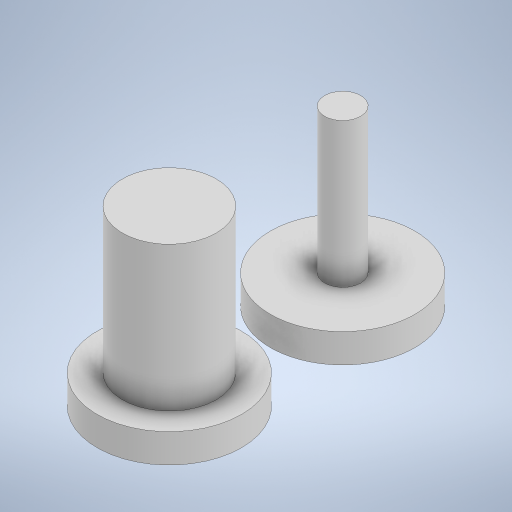
# Autodesk Inventor part: V3_O1
Saved by Autodesk Inventor 2023.1 (Build 271208000, 208)
## iProperties
Created: 2023-04-22
Part Number: V3_O1
Material: Generisch
Document SubType Name: Sheet Metal
Designer: marco
Density: 1 g/cm^3
Sheet Metal Rule: Standard_mm
Appearance: Vorgabe
Author: marco
Autodesk Inventor part; units mm, degrees
ref_plane "YZ Plane" through (0, 0, 0) normal (1, 0, 0) x (0, 1, 0)
ref_plane "XZ Plane" through (0, 0, 0) normal (0, 1, 0) x (-1, 0, 0)
ref_plane "XY Plane" through (0, 0, 0) normal (0, 0, 1) x (1, 0, 0)
sketch "Skizze1" plane through (0, 0, 0) normal (0, 1, 0) x (-1, 0, 0)
  circle A0 centre (0, 0) radius 2.5
  dimension "d0" = 5
  constraints: 1 centre point, 1 coincident
  measures "d0" diameter of A0
extrude "Extrusion1" add sketch "Skizze1" along normal blind 1
sketch "Skizze2" plane through (0, 1, 0) normal (0, 1, 0) x (1, 0, 0)
  circle A0 centre (0, 0) radius 2.5 projected
  circle A1 centre (0, 0) radius 0.5
  dimension "d3" = 1
  constraints: 1 centre point, 1 coincident
  measures "d3" diameter of A1
extrude "Extrusion2" add sketch "Skizze2" along normal blind 7.4 contours A1
thicken "Verdickung1" operation cut thickness 4 both sides no extend neighbours no toward (0, -1, 0) faces at (0.3086, 8.4, 0.1558)
thicken "Verdickung2" operation cut thickness 1.4 both sides no extend neighbours no toward (0, -1, 0) faces at (0.3086, 4.4, 0.1558)
thicken "Verdickung3" operation add thickness 0.125 both sides no extend neighbours no toward (0.9967573, 0, 0.0804666) faces at (0.4984, 1.6667, 0.0402)
thicken "Verdickung4" operation add thickness 1 both sides no extend neighbours no toward (0, 1, 0) faces at (0.4826, 3, -0.0333)
sketch "Skizze3" plane through (0, 0, 0) normal (0, -1, 0) x (1, 0, 0)
  circle A0 centre (0, 6) radius 2.5
  point P0 (0, 0)
  dimension "d14" = 5
  dimension "d15" = 6
  constraints: 1 centre point
  measures "d14" diameter of A0
  measures "d15" distance of A0.centre point (0, 0)
extrude "Extrusion3" add sketch "Skizze3" against normal blind 1
sketch "Skizze4" plane through (0, 1, 6) normal (0, 1, 0) x (1, 0, 0)
  circle A0 centre (0, 0) radius 2.5 projected
  circle A1 centre (0, 0) radius 1.625
  point P0 (0, 6)
  dimension "d18" = 3.25
  constraints: 1 centre point, 1 coincident
  measures "d18" diameter of A1
extrude "Extrusion4" add sketch "Skizze4" along normal blind 5 contours A1
thicken "Verdickung5" operation add thickness 2 both sides no extend neighbours no toward (0, 1, 0) faces at (0.4826, 4, -0.0333)
equation "\"Biegeradius\" = Stärke"
equation "\"BreiteBiegungsfreistellung\" = Stärke"
equation "\"TiefeBiegungsfreistellung\" = 0.5 * Stärke"
equation "\"GrößeEckenfreistellung\" = 4 * Stärke"
equation "\"MinimalRest\" = 2 * Stärke"
equation "\"Übergangsradius\" = Biegeradius"
equation "\"JacobiRadiusGröße\" = Biegeradius"
equation "\"Abstandsgröße\" = Stärke"
equation "\"Stärke\" = 0.5"
